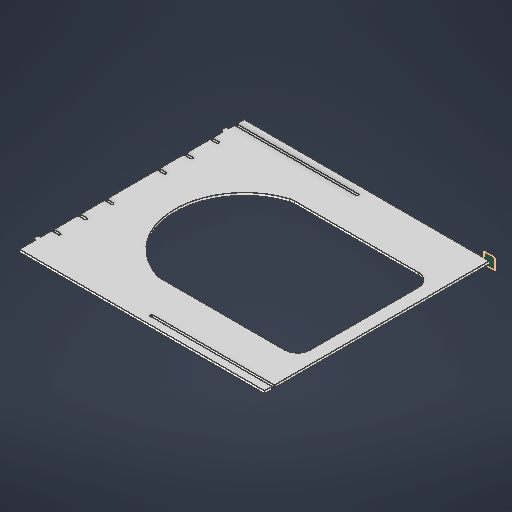
# Autodesk Inventor part: outside_leg
Saved by Autodesk Inventor 2027.1 (Build 311270010, 270A)
## iProperties
Created: 2025-09-11
Part Number: outside_leg
Material: Foam Core Board
Document SubType Name: Modeling
Designer: Nick
Density: 0.141998 g/cm^3
Appearance: Default(1)
Mass: 86.0449 g
Surface Area: 2632.14 cm^2
Volume: 605.959 cm^3
Author: Nick
Autodesk Inventor part; units mm, degrees
ref_plane "YZ Plane" through (0, 0, 0) normal (1, 0, 0) x (0, 1, 0)
ref_plane "XZ Plane" through (0, 0, 0) normal (0, 1, 0) x (-1, 0, 0)
ref_plane "XY Plane" through (0, 0, 0) normal (0, 0, 1) x (1, 0, 0)
sketch "Sketch1" plane through (0, 0, 0) normal (0, 1, 0) x (-1, 0, 0)
  line L0 (0, 0) -> (485, 0)
  line L1 (485, 0) -> (485, -415)
  line L2 (485, -415) -> (0, -415)
  line L3 (0, -415) -> (0, 0)
  line L4 (0, 0) -> (25, 0)
  line L5 (25, 0) -> (25, -415)
  line L6 (25, -415) -> (0, -415)
  line L7 (0, -415) -> (0, 0)
  line L8 (25, 0) -> (300, 0)
  line L9 (300, 0) -> (300, -75)
  line L10 (300, -75) -> (25, -75)
  line L11 (25, -75) -> (25, 0)
  line L12 (25, -415) -> (300, -415)
  line L13 (300, -415) -> (300, -340)
  line L14 (300, -340) -> (25, -340)
  line L15 (25, -340) -> (25, -415)
  line L16 (25, -207.5) -> (400, -207.5)
  arc A0 (300, -340) -> (300, -75) centre (262.2188, -207.5) ccw
  point P0 (25, -340)
  point P1 (25, -75)
  dimension "d0" = 485
  dimension "d1" = 415
  dimension "d2" = 25
  dimension "d3" = 275
  dimension "d4" = 75
  dimension "d5" = 275
  dimension "d6" = 75
  dimension "d7" = 375
  constraints: 34 end point, 8 parallel, 5 horizontal, 4 perpendicular, 3 point on circle, 1 centre point, 1 midpoint, 1 point on line
  measures "d0" distance of L1.end L2.end
  measures "d1" distance of L0.end L1.end
  measures "d2" distance of L5.end L6.end
  measures "d3" distance of L9.end L10.end
  measures "d4" distance of L8.end L9.end
  measures "d5" distance of L14.end L13.end
  measures "d6" distance of L13.end L12.end
  measures "d7" distance of L16.start L16.end
extrude "Extrusion1" add sketch "Sketch1" along normal blind 5 contours L0 L5 L2 L3 | L0 L9 L10 L5 | L0 L1 L2 L13 A0 L9 | L5 L14 L13 L2
fillet "Fillet1" radius 25 4 edges at (-25, 2.5, -340) (-25, 2.5, -75) (-300, 2.5, -75) (-300, 2.5, -340)
sketch "Sketch2" plane through (-485, 0, 0) normal (0, 0, 1) x (1, 0, 0)
  line L0 (0, 0) -> (485, 0) projected
  line L1 (0, 5) -> (485, 5) projected
  line L2 (0, 0) -> (485, 0)
  line L3 (485, 0) -> (485, 5)
  line L4 (485, 5) -> (0, 5)
  line L5 (0, 5) -> (0, 0)
  constraints: 8 end point, 2 parallel, 1 horizontal, 1 perpendicular
extrude "Extrusion2" add sketch "Sketch2" along normal blind 10
sketch "Sketch3" plane through (0, 0, -415) normal (0, 0, -1) x (-1, 0, 0)
  line L0 (485, 0) -> (485, 5) projected
  line L1 (485, 5) -> (0, 5)
  line L2 (0, 5) -> (0, 0)
  line L3 (0, 0) -> (485, 0)
  line L4 (485, 0) -> (485, 5)
  constraints: 8 end point, 2 parallel, 1 horizontal, 1 perpendicular
extrude "Extrusion3" add sketch "Sketch3" along normal blind 10
sketch "Sketch4" plane through (0, 5, 0) normal (0, 1, 0) x (1, 0, 0)
  line L0 (0, 0) -> (-242.5, 0)
  line L1 (-242.5, 0) -> (-242.5, 4.5)
  line L2 (-242.5, 4.5) -> (0, 4.5)
  line L3 (0, 4.5) -> (0, 0)
  line L4 (-485, -10) -> (-485, 425) projected
  line L5 (-485, 425) -> (-485, 415)
  line L6 (-485, 415) -> (-242.5, 415)
  line L7 (-242.5, 415) -> (-242.5, 410.5)
  line L8 (-242.5, 410.5) -> (-485, 410.5)
  line L9 (-485, 410.5) -> (-485, 415)
  line L10 (0, 425) -> (0, -10) projected
  dimension "d15" = 4.5
  dimension "d16" = 4.5
  dimension "d17" = 242.5
  dimension "d18" = 10
  dimension "d19" = 4.5
  dimension "d20" = 242.5
  constraints: 18 end point, 4 parallel, 2 horizontal, 2 perpendicular, 1 point on line
  measures "d15" distance of L0.end L1.end
  measures "d16" distance between parallel lines of L0 L2
  measures "d17" distance between parallel lines of L4 L1
  measures "d18" distance of L4.end L5.end
  measures "d19" distance of L6.end L7.end
  measures "d20" distance between parallel lines of L10 L7
extrude "Extrusion4" cut sketch "Sketch4" against normal blind 5
sketch "Sketch6" plane through (0, 5, 0) normal (0, 1, 0) x (1, 0, 0)
  line L0 (-485, 410.5) -> (-485, 202.5446)
  line L1 (-485, 410.5) -> (-485, 362)
  line L2 (-485, 362) -> (-470, 362)
  line L3 (-470, 362) -> (-470, 366.5)
  line L4 (-470, 366.5) -> (-485, 366.5)
  line L5 (-485, 366.5) -> (-485, 362)
  line L6 (-485, 309.75) -> (-470, 309.75)
  line L7 (-470, 309.75) -> (-470, 314.25)
  line L8 (-470, 314.25) -> (-485, 314.25)
  line L9 (-485, 314.25) -> (-485, 309.75)
  line L10 (-485, 257.5) -> (-470, 257.5)
  line L11 (-470, 257.5) -> (-470, 262)
  line L12 (-470, 262) -> (-485, 262)
  line L13 (-485, 262) -> (-485, 257.5)
  line L14 (-485, 205.25) -> (-470, 205.25)
  line L15 (-470, 205.25) -> (-470, 209.75)
  line L16 (-470, 209.75) -> (-485, 209.75)
  line L17 (-485, 209.75) -> (-485, 205.25)
  line L18 (-485, 153) -> (-470, 153)
  line L19 (-470, 153) -> (-470, 157.5)
  line L20 (-470, 157.5) -> (-485, 157.5)
  line L21 (-485, 157.5) -> (-485, 153)
  line L22 (-485, 100.75) -> (-470, 100.75)
  line L23 (-470, 100.75) -> (-470, 105.25)
  line L24 (-470, 105.25) -> (-485, 105.25)
  line L25 (-485, 105.25) -> (-485, 100.75)
  line L26 (-485, 48.5) -> (-470, 48.5)
  line L27 (-470, 48.5) -> (-470, 53)
  line L28 (-470, 53) -> (-485, 53)
  line L29 (-485, 53) -> (-485, 48.5)
  line L30 (-485, -10) -> (-485, 410.5) projected
  line L31 (-485, 410.5) -> (-452.1188, 410.5)
  line L32 (-242.5, 410.5) -> (-485, 410.5) projected
  point P0 (0, 0)
  dimension "d27" = 48.5
  dimension "d28" = 15
  dimension "d29" = 4.5
  dimension "d30" = 52.25
  dimension "d32" = 0
  constraints: 62 end point, 2 parallel, 2 point on line, 1 horizontal, 1 perpendicular, 1 vertical, 48 other
  measures "d27" distance of L1.start L1.end
  measures "d28" distance of L4.end L3.end
  measures "d29" distance of L3.end L3.start
  measures "d30" distance of L1.end L9.end
  measures "d32" distance between parallel lines of L30 L29
extrude "Extrusion5" cut sketch "Sketch6" against normal blind 5 contours L4 L3 L2 L0 | L28 L27 L26 L29 | L24 L23 L22 L25 | L20 L19 L18 L21 | L12 L11 L10 L0 | L8 L7 L6 L0
ref_plane "Work Plane1" through (0, 5, -430.1373) normal (0, 0, -1) x (-1, 0, 0)
fillet "Fillet2" radius 1 32 edges at (-242.5, 2.5, 0) (-242.5, 2.5, -4.5) (0, 2.5, 0) (0, 2.5, -4.5) (-470, 2.5, -48.5) (-470, 2.5, -53) (-485, 2.5, -53) (-485, 2.5, -48.5) (-470, 2.5, -100.75) (-470, 2.5, -105.25) (-485, 2.5, -105.25) (-485, 2.5, -100.75) (-485, 2.5, -157.5) (-485, 2.5, -153) (-470, 2.5, -153) (-470, 2.5, -157.5) (-485, 2.5, -257.5) (-470, 2.5, -257.5) (-470, 2.5, -262) (-485, 2.5, -262) (-470, 2.5, -309.75) (-470, 2.5, -314.25) (-485, 2.5, -314.25) (-485, 2.5, -309.75) (-485, 2.5, -366.5) (-485, 2.5, -362) (-470, 2.5, -362) (-470, 2.5, -366.5) (-485, 2.5, -410.5) (-485, 2.5, -415) (-242.5, 2.5, -410.5) (-242.5, 2.5, -415)
sketch "Sketch10" plane through (-485, 0, -409.5) normal (-1, 0, 0) x (0, 0, 1)
  line L0 (42, 5) -> (0, 5) projected
  line L1 (21, 5) -> (21, 0)
  line L2 (21, 0) -> (11, 0)
  line L3 (0, 0) -> (42, 0) projected
  line L4 (11, 0) -> (31, 0)
  line L5 (31, 0) -> (31, 5)
  line L6 (31, 5) -> (11, 5)
  line L7 (11, 5) -> (11, 0)
  line L8 (70.6707, 5) -> (333.3293, 5) projected
  line L9 (202, 5) -> (202, -36.8909)
  line L10 (383, 5) -> (383, 0)
  line L11 (383, 0) -> (393, 0)
  line L12 (393, 0) -> (373, 0)
  line L13 (373, 0) -> (373, 5)
  line L14 (373, 5) -> (393, 5)
  line L15 (393, 5) -> (393, 0)
  point P0 (409.5, 0)
  point P1 (31, 0)
  point P2 (11, 5)
  dimension "d44" = 10
  dimension "d45" = 20
  constraints: 26 end point, 6 symmetric about line, 2 midpoint, 2 parallel, 2 point on line, 2 vertical, 1 horizontal, 1 perpendicular
  measures "d44" distance of L1.end L2.end
  measures "d45" distance of L6.end L5.end
extrude "Extrusion9" add sketch "Sketch10" along normal blind 5 contours L1 L2 L7 L0 | L14 L15 L11 L10
sketch "Sketch12" plane through (0, 5, 0) normal (0, 1, 0) x (1, 0, 0)
  line L0 (0, -10) -> (-485, -10)
  line L1 (-485, -10) -> (-485, -15)
  line L2 (-485, -15) -> (0, -15)
  line L3 (0, -15) -> (0, -10)
  line L4 (0, 425) -> (-485, 425) projected
  line L5 (-485, 425) -> (0, 425)
  line L6 (0, 425) -> (0, 430)
  line L7 (0, 430) -> (-485, 430)
  line L8 (-485, 430) -> (-485, 425)
  point P0 (0, 0)
  dimension "d48" = 5
  dimension "d49" = 5
  constraints: 16 end point, 4 parallel, 2 horizontal, 2 perpendicular, 1 point on line
  measures "d48" distance of L1.end L0.end
  measures "d49" distance of L6.end L5.end
extrude "Extrusion10" add sketch "Sketch12" against normal blind 5
body "Solid1"
